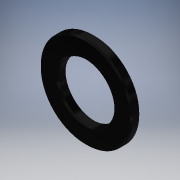
# Autodesk Inventor part: thrust washer
Saved by Autodesk Inventor 2019 (Build 230136000, 136)
## iProperties
Shininess: 41.0
Length Units: 11272
Angle Units: 11279
Time Units: 11290
Mass Units: 11286
Length Display Precision: 3
Angle Display Precision: 2
Compacted: True
Created: 2001-07-10
Part Number: thrust washer
Document SubType Name: Modeling
Designer: Autodesk, Inc.
Mass: 0.0226787 g
Surface Area: 0.887749 cm^2
Volume: 0.0243857 cm^3
Density: 0.93 g/cm^3
Material: Rubber
Appearance: Glossy - Black
Density: 0.0
Volumn: 0.0
Area: 0.0
PropertySet Name: Model Information
Control State: 0
Master: False
Checked Out: False
Author: Autodesk, Inc.
Autodesk Inventor part; units mm, degrees
ref_plane "YZ Plane" through (0, 0, 0) normal (1, 0, 0) x (0, 1, 0)
ref_plane "XZ Plane" through (0, 0, 0) normal (0, 1, 0) x (-1, 0, 0)
ref_plane "Work Plane1" through (0, 0, 0) normal (0, 0, 1) x (1, 0, 0)
sketch "Sketch2" plane through (0, 0, 0) normal (0, 0, 1) x (1, 0, 0)
  arc A0 (-2.0996, 1.5875) -> (1.4502, 1.5875) centre (-0.3247, 0) ccw projected
  circle A1 centre (-0.3247, 0) radius 2.3813
  circle A2 centre (-0.3247, 0) radius 3.9633
  constraints: 2 coincident, 1 centre point, 4 other
extrude "Extrusion1" add sketch "Sketch2" along normal blind 0.7937
chamfer "Chamfer1" distance 0.127 angle 45 4 edges at (-4.288, 0, 0) (-4.288, 0, 0.7937) (-2.706, 0, 0.7937) (-2.706, 0, 0)
body "Solid1"
